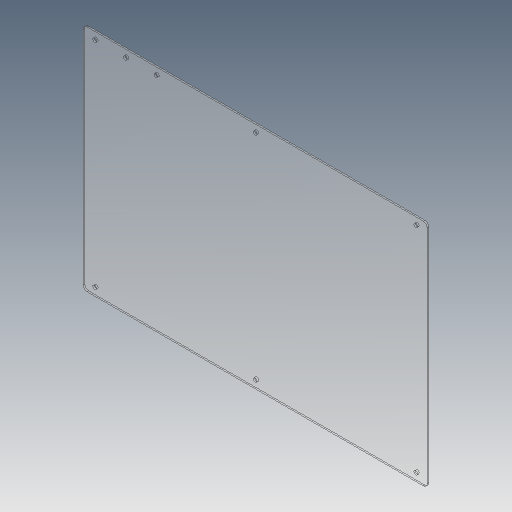
# Autodesk Inventor part: 防水2
Saved by Autodesk Inventor 2020.3 (Build 243373000, 373)
## iProperties
Part Number: 防水2
Material: PET プラスチック
Document SubType Name: Modeling
Designer: highs
Density: 1.541 g/cm^3
Appearance: ポリカーボネート - クリア
Author: highs
Autodesk Inventor part; units mm, degrees
ref_plane "YZ Plane" through (0, 0, 0) normal (1, 0, 0) x (0, 1, 0)
ref_plane "XZ Plane" through (0, 0, 0) normal (0, 1, 0) x (-1, 0, 0)
ref_plane "XY Plane" through (0, 0, 0) normal (0, 0, 1) x (1, 0, 0)
sketch "スケッチ1" plane through (0, 0, 0) normal (0, 0, 1) x (1, 0, 0)
  line L0 (0, 0) -> (450, 0)
  line L1 (450, 0) -> (450, 300)
  line L2 (450, 300) -> (0, 300)
  line L3 (0, 300) -> (0, 0)
  line L4 (10, 290) -> (440, 290) construction
  line L5 (440, 290) -> (440, 10) construction
  line L6 (440, 10) -> (10, 10) construction
  line L7 (10, 10) -> (10, 290) construction
  circle A0 centre (15, 290) radius 2.5
  circle A1 centre (435, 290) radius 2.5
  circle A2 centre (225, 290) radius 2.5
  circle A3 centre (15, 10) radius 2.5
  circle A4 centre (435, 10) radius 2.5
  line L8 (225, 0) -> (225, 10) construction
  line L9 (225, 287.5) -> (225, 300) construction
  circle A5 centre (225, 10) radius 2.5
  circle A6 centre (55, 290) radius 2.5
  circle A7 centre (95, 290) radius 2.5
  dimension "d0" = 450
  dimension "d1" = 300
  dimension "d2" = 10
  dimension "d3" = 15
  dimension "d4" = 15
  dimension "d5" = 5
  dimension "d9" = 5
  dimension "d10" = 15
  dimension "d12" = 15
  dimension "d16" = 40
  dimension "d17" = 40
  constraints: 20 end point, 7 centre point, 6 point on line, 5 equal radius, 4 midpoint, 4 parallel, 2 perpendicular, 1 coincident, 1 horizontal, 1 vertical, 1 vertical alignment, 6 other
  measures "d0" distance of L0.start L0.end
  measures "d1" distance of L2.end L0.start
  measures "d2" distance between parallel lines of L2 L4
  measures "d3" distance from line of L3 A0.centre
  measures "d4" distance from line of L1 A1.centre
  measures "d5" diameter of A0
  measures "d9" diameter of A3
  measures "d10" distance from line of L3 A3.centre
  measures "d12" distance from line of L1 A4.centre
  measures "d16" distance of A7.centre A6.centre
  measures "d17" distance of A6.centre A0.centre
extrude "押し出し1" add sketch "スケッチ1" along normal blind 2
fillet "フィレット1" radius 5 4 edges at (450, 0, 1) (450, 300, 1) (0, 0, 1) (0, 300, 1)
